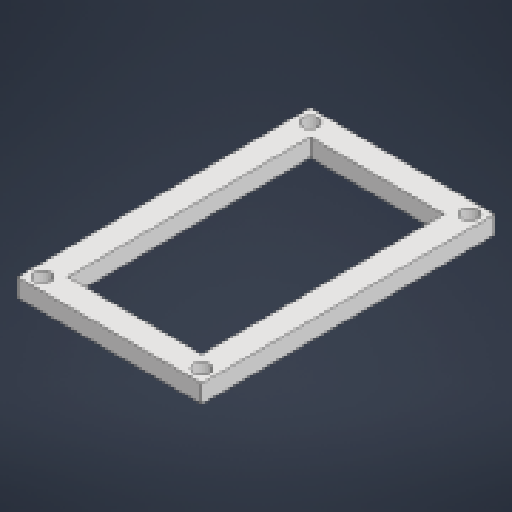
# Autodesk Inventor part: PCB_Housing_06_V4
Saved by Autodesk Inventor 2026.2 (Build 302298000, 298)
## iProperties
Created: 2026-03-17
Part Number: PCB_Housing_06_V4
Material: Generic
Document SubType Name: Modeling
Designer: vckot
Density: 1 g/cm^3
Appearance: Default
Author: vckot
Autodesk Inventor part; units mm, degrees
ref_plane "YZ Plane" through (0, 0, 0) normal (1, 0, 0) x (0, 1, 0)
ref_plane "XZ Plane" through (0, 0, 0) normal (0, 1, 0) x (-1, 0, 0)
ref_plane "XY Plane" through (0, 0, 0) normal (0, 0, 1) x (1, 0, 0)
sketch "Sketch1" plane through (0, 0, 0) normal (0, 1, 0) x (-1, 0, 0)
  line L0 (22, -37) -> (-22, -37) construction
  line L1 (-22, -37) -> (-22, 37) construction
  line L2 (-22, 37) -> (22, 37) construction
  line L3 (22, 37) -> (22, -37) construction
  line L4 (22, -37) -> (-22, 37) construction
  line L5 (-22, -37) -> (22, 37) construction
  line L6 (-19, -34) -> (19, -34)
  line L7 (19, -34) -> (19, 34)
  line L8 (19, 34) -> (-19, 34)
  line L9 (-19, 34) -> (-19, -34)
  line L10 (-25.5, -40.5) -> (25.5, -40.5)
  line L11 (25.5, -40.5) -> (25.5, 40.5)
  line L12 (25.5, 40.5) -> (-25.5, 40.5)
  line L13 (-25.5, 40.5) -> (-25.5, -40.5)
  point P0 (0, 0)
  dimension "d0" = 44
  dimension "d1" = 74
  dimension "d2" = 3
  dimension "d3" = 3.5
  constraints: 28 end point, 6 parallel, 3 coincident, 3 perpendicular, 2 midpoint, 1 horizontal, 6 other
  measures "d0" distance of L1.end L2.end
  measures "d1" distance of L0.end L1.end
  measures "d2" distance between parallel lines of L0 L6
  measures "d3" distance between parallel lines of L0 L10
extrude "Extrusion1" add sketch "Sketch1" against normal blind 5
hole "Hole1" at (22, 0, -37) at (-22, 0, -37) at (-22, 0, 37) at (22, 0, 37) direction (0, -1, 0) diameter 4.5 end through all
sketch "Sketch2" plane through (0, 0, 0) normal (0, 1, 0) x (1, 0, 0)
  line L0 (19, -34) -> (25.5, -34)
  line L1 (25.5, -34) -> (25.5, -40.5)
  line L2 (25.5, -40.5) -> (19, -40.5)
  line L3 (19, -40.5) -> (19, -34)
  line L4 (25.5, -40.5) -> (-25.5, -40.5) projected
  line L5 (-19, -34) -> (-25.5, -34)
  line L6 (-25.5, -34) -> (-25.5, -40.5)
  line L7 (-25.5, -40.5) -> (-19, -40.5)
  line L8 (-19, -40.5) -> (-19, -34)
  line L9 (19, 34) -> (-19, 34) projected
  line L10 (-25.5, 40.5) -> (25.5, 40.5) projected
  line L11 (-19, 34) -> (-25.5, 34)
  line L12 (-25.5, 34) -> (-25.5, 40.5)
  line L13 (-25.5, 40.5) -> (-19, 40.5)
  line L14 (-19, 40.5) -> (-19, 34)
  line L15 (19, 34) -> (25.5, 34)
  line L16 (25.5, 34) -> (25.5, 40.5)
  line L17 (25.5, 40.5) -> (19, 40.5)
  line L18 (19, 40.5) -> (19, 34)
  circle A0 centre (22, -37) radius 2.25 projected
  circle A1 centre (-22, -37) radius 2.25 projected
  circle A2 centre (-22, 37) radius 2.25 projected
  circle A3 centre (22, 37) radius 2.25 projected
  point P0 (0, 0)
  constraints: 32 end point, 8 parallel, 4 horizontal, 4 perpendicular
extrude "Extrusion2" [suppressed]
body "Solid1"
